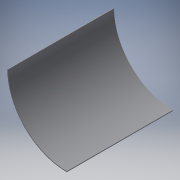
# Autodesk Inventor part: Part90
Saved by Autodesk Inventor 2016 (Build 200138000, 138)
## iProperties
Created: 2016-09-04
Part Number: Part90
Material: Generic
Document SubType Name: Modeling
Designer: gus
Density: 1 g/cm^3
Appearance: Default
Author: gus
Autodesk Inventor part; units mm, degrees
ref_plane "YZ Plane" through (0, 0, 0) normal (1, 0, 0) x (0, 1, 0)
ref_plane "XZ Plane" through (0, 0, 0) normal (0, 1, 0) x (-1, 0, 0)
ref_plane "XY Plane" through (0, 0, 0) normal (0, 0, 1) x (1, 0, 0)
sketch "Sketch1" plane through (0, 0, 0) normal (0, 0, 1) x (1, 0, 0)
  arc A0 (0, 0) -> (190.5, -190.5) centre (190.5, 0) ccw
  line L0 (0, 0) -> (190.5, 0) construction
  line L1 (190.5, 0) -> (190.5, -190.5) construction
  arc A1 (3.175, 0) -> (190.5, -187.325) centre (190.5, 0) ccw
  line L2 (3.175, 0) -> (0, 0)
  line L3 (190.5, -190.5) -> (190.5, -187.325)
  dimension "d0" = 190.5
  dimension "d1" = 3.175
  constraints: 8 end point, 4 point on circle, 2 centre point, 2 perpendicular, 2 point on line, 1 collinear, 1 concentric, 1 horizontal
  measures "d0" distance of L0.start L0.end
  measures "d1" radial gap between concentric circles of A1 A0
extrude "Extrusion1" add sketch "Sketch1" against normal blind 384.175
body "Solid1"
